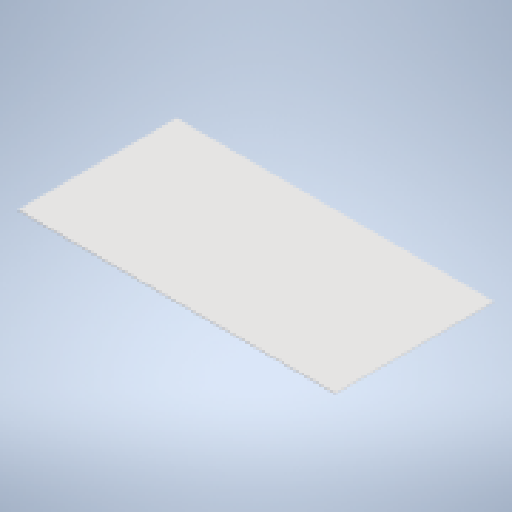
# Autodesk Inventor part: TableroMadera
Saved by Autodesk Inventor 2024 (Build 280153000, 153)
## iProperties
Created: 2024-07-25
Part Number: TableroMadera
Material: Genérico
Document SubType Name: Modeling
Designer: sergi
Density: 1 g/cm^3
Appearance: Valor por defecto
Author: sergi
Autodesk Inventor part; units mm, degrees
ref_plane "YZ Plane" through (0, 0, 0) normal (1, 0, 0) x (0, 1, 0)
ref_plane "XZ Plane" through (0, 0, 0) normal (0, 1, 0) x (-1, 0, 0)
ref_plane "XY Plane" through (0, 0, 0) normal (0, 0, 1) x (1, 0, 0)
sketch "Boceto1" plane through (0, 0, 0) normal (0, 1, 0) x (-1, 0, 0)
  line L0 (-600, -300) -> (600, -300)
  line L1 (600, -300) -> (600, 300)
  line L2 (600, 300) -> (-600, 300)
  line L3 (-600, 300) -> (-600, -300)
  line L4 (-600, -300) -> (600, 300) construction
  line L5 (600, -300) -> (-600, 300) construction
  point P0 (0, 0)
  dimension "d0" = 1200
  dimension "d1" = 600
  constraints: 12 end point, 2 midpoint, 2 parallel, 1 horizontal, 1 perpendicular
  measures "d0" distance of L2.end L1.end
  measures "d1" distance of L1.end L0.end
extrude "Extrusión1" add sketch "Boceto1" along normal blind 3
